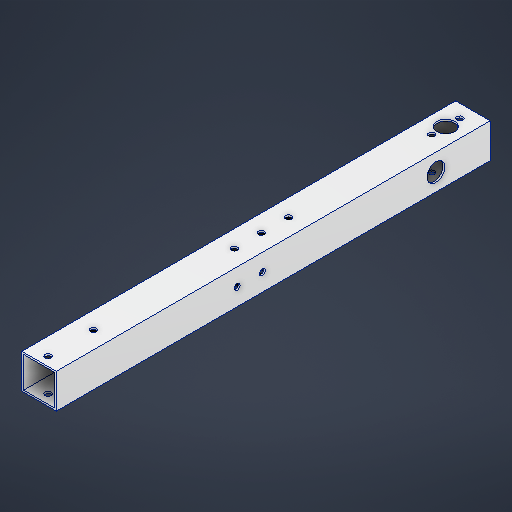
# Autodesk Inventor part: perfil
Saved by Autodesk Inventor 2026.1 (Build 301233020, 233B)
## iProperties
Created: 2025-07-22
Part Number: perfil
Material: Aluminio 6061
Document SubType Name: Modeling
Designer: rodri
Density: 2.7 g/cm^3
Appearance: Aluminio - Plano
Mass: 46.0498 g
Surface Area: 345.109 cm^2
Volume: 17.0555 cm^3
Author: rodri
Autodesk Inventor part; units mm, degrees
ref_plane "YZ Plane" through (0, 0, 0) normal (1, 0, 0) x (0, 1, 0)
ref_plane "XZ Plane" through (0, 0, 0) normal (0, 1, 0) x (-1, 0, 0)
ref_plane "XY Plane" through (0, 0, 0) normal (0, 0, 1) x (1, 0, 0)
sketch "Boceto1" plane through (0, 0, 0) normal (0, 0, 1) x (1, 0, 0)
  line L0 (-9.55, -9.55) -> (9.55, -9.55)
  line L1 (9.55, -9.55) -> (9.55, 9.55)
  line L2 (9.55, 9.55) -> (-9.55, 9.55)
  line L3 (-9.55, 9.55) -> (-9.55, -9.55)
  line L4 (-9.55, -9.55) -> (9.55, 9.55) construction
  line L5 (9.55, -9.55) -> (-9.55, 9.55) construction
  line L6 (-8.55, 8.55) -> (8.55, 8.55)
  line L7 (8.55, 8.55) -> (8.55, -8.55)
  line L8 (8.55, -8.55) -> (-8.55, -8.55)
  line L9 (-8.55, -8.55) -> (-8.55, 8.55)
  point P0 (0, 0)
  dimension "d0" = 19.1
  dimension "d1" = 19.1
  dimension "d2" = 1
  constraints: 20 end point, 4 parallel, 2 midpoint, 2 perpendicular, 1 horizontal, 3 other
  measures "d0" distance of L0.end L1.end
  measures "d1" distance of L1.end L2.end
  measures "d2" distance between parallel lines of L2 L6
extrude "Extrusión1" add sketch "Boceto1" against normal blind 240
sketch "Boceto2" plane through (-9.55, 9.55, 0) normal (0, 1, 0) x (1, 0, 0)
  line L0 (19.1, 0) -> (0, 0) projected
  line L1 (9.55, 0) -> (9.55, 240) construction
  line L2 (19.1, 240) -> (0, 240) construction
  point P0 (9.55, 5)
  point P1 (9.55, 30)
  point P2 (9.55, 108)
  point P3 (9.55, 123)
  point P4 (9.55, 138)
  point P5 (9.55, 225)
  point P6 (9.55, 232.75)
  point P7 (9.55, 217.25)
  dimension "d5" = 5
  dimension "d6" = 30
  dimension "d7" = 78
  dimension "d10" = 15
  dimension "d15" = 15
  dimension "d19" = 15.5
  dimension "d24" = 7.75
  constraints: 2 end point, 2 point on line, 2 vertical, 1 midpoint, 3 other
  measures "d5" distance from line of point (9.55, 5) L0
  measures "d6" distance from line of point (9.55, 30) L0
  measures "d7" distance of point (9.55, 108) point (9.55, 30)
  measures "d10" distance of point (9.55, 108) point (9.55, 123)
  measures "d15" distance from line of point (9.55, 225) L2
  measures "d19" distance of point (9.55, 232.75) point (9.55, 217.25)
  measures "d24" distance of point (9.55, 232.75) point (9.55, 225)
hole "Agujero1" at (0, 9.55, -5) at (0, 9.55, -30) at (0, 9.55, -108) at (0, 9.55, -123) at (0, 9.55, -138) at (0, 9.55, -217.25) at (0, 9.55, -232.75) direction (0, -1, 0) diameter 3.4 end through all clearance for "Tornillo para maquinaria de cabeza plana" size "M3" standard "Perfil M métrico ANSI"
hole "Agujero2" at (0, 9.55, -225) direction (0, -1, 0) diameter 10 depth 1
sketch "Boceto3" plane through (9.55, -9.55, 0) normal (1, 0, 0) x (0, 0, -1)
  line L0 (240, 19.1) -> (240, 0) construction
  line L1 (240, 9.55) -> (210, 9.55) construction
  circle A0 centre (210, 9.55) radius 5
  point P0 (0, 9.55)
  dimension "d39" = 30
  dimension "d40" = 10
  constraints: 2 end point, 1 centre point, 1 coincident, 1 horizontal, 1 midpoint
  measures "d39" distance of L1.start L1.end
  measures "d40" diameter of A0
extrude "Extrusión2" cut sketch "Boceto3" against normal up to next
sketch "Boceto4" plane through (9.55, -9.55, 0) normal (1, 0, 0) x (0, 0, -1)
  line L0 (0, 9.55) -> (191.9692, 9.55) construction
  line L1 (0, 0) -> (0, 19.1) construction
  point P0 (100, 9.55)
  point P1 (114, 9.55)
  dimension "d43" = 100
  dimension "d44" = 14
  constraints: 2 end point, 2 point on line, 1 horizontal
  measures "d43" distance from line of point (100, 9.55) L1
  measures "d44" distance of point (114, 9.55) point (100, 9.55)
hole "Agujero3" at (9.55, 0, -100) at (9.55, 0, -114) direction (-1, 0, 0) diameter 3.4 end through all clearance for "Tornillo para maquinaria de cabeza plana" size "M3" standard "Perfil M métrico ANSI"
